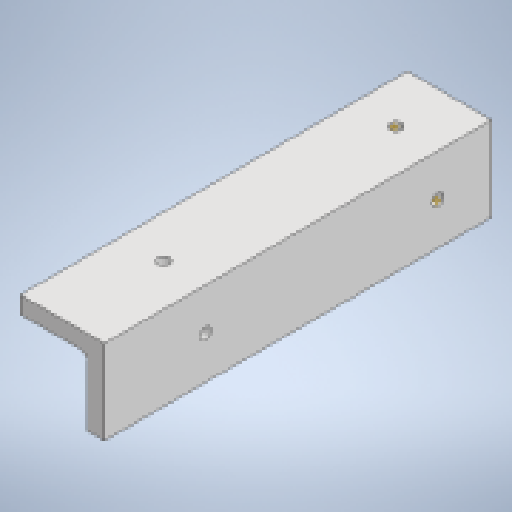
# Autodesk Inventor part: wall-joint
Saved by Autodesk Inventor 2023 (Build 270158000, 158)
## iProperties
Created: 2022-10-04
Part Number: wall-joint
Material: Generic
Document SubType Name: Modeling
Designer: carso
Density: 1 g/cm^3
Appearance: Default
Author: carso
Autodesk Inventor part; units mm, degrees
ref_plane "YZ Plane" through (0, 0, 0) normal (1, 0, 0) x (0, 1, 0)
ref_plane "XZ Plane" through (0, 0, 0) normal (0, 1, 0) x (-1, 0, 0)
ref_plane "XY Plane" through (0, 0, 0) normal (0, 0, 1) x (1, 0, 0)
sketch "Sketch1" plane through (0, 0, 0) normal (0, 1, 0) x (-1, 0, 0)
  line L0 (0, 0) -> (0, 115)
  line L1 (0, 115) -> (5, 115)
  line L2 (0, 0) -> (25, 0)
  line L3 (25, 0) -> (25, 2)
  line L4 (5, 115) -> (5, 0)
  line L5 (25, 2) -> (0, 2)
  line L6 (5, 2) -> (10, 2)
  line L7 (5, 7) -> (5, 2)
  dimension "d1" = 5
  dimension "d2" = 25
  dimension "d3" = 2
  dimension "d60" = 115
  constraints: 16 end point, 4 point on line, 3 perpendicular, 2 horizontal, 2 vertical
  measures "d1" distance of L0.end L1.end
  measures "d2" distance of L0.start L2.end
  measures "d3" distance of L2.end L3.end
  measures "d60" distance of L0.start L0.end
extrude "Extrusion2" add sketch "Sketch1" along normal blind 20
sketch "Sketch3" plane through (0, 20, 0) normal (0, 1, 0) x (1, 0, 0)
  line L0 (0, 0) -> (-25, 0)
  line L1 (-25, 0) -> (-25, -2) projected
  line L2 (-25, 0) -> (-25, -2)
  line L3 (-25, -2) -> (-5, -2)
  line L4 (-5, -115) -> (0, -115) projected
  line L5 (-5, -115) -> (0, -115)
  line L6 (0, 0) -> (-25, 0) projected
  line L7 (0, -115) -> (0, 0)
  line L8 (-5, -115) -> (-25, -115)
  line L9 (-25, -115) -> (-25, -2)
  constraints: 14 end point, 3 perpendicular, 2 collinear, 2 horizontal
extrude "Extrusion3" add sketch "Sketch3" along normal blind 5
fillet "Face Fillet1" radius 2 1 edges at (-5, 10, 2)
fillet "Face Fillet2" radius 2 1 edges at (-16, 20, 2)
hole "Hole3" at (0, 12.5, 15.9996) direction (-1, 0, 0) diameter 3.5 depth 8.8
hole "Hole4" at (-12.5, 25, 16) direction (0, -1, 0) diameter 3.5 depth 8.8
sketch "Sketch11" plane through (0, 25, 0) normal (0, 1, 0) x (1, 0, 0)
  line L0 (-5, -115) -> (0, -115) projected
  line L1 (0, -115) -> (-12.5, -115)
  line L2 (-12.5, -115) -> (-12.5, -85)
  line L3 (-12.5, -85) -> (0, -85)
  line L4 (0, -85) -> (0, -115)
  point P0 (0, 0)
  dimension "d82" = 12.5
  dimension "d83" = 30
  constraints: 8 end point, 2 parallel, 1 horizontal, 1 perpendicular
  measures "d82" distance of L2.end L3.end
  measures "d83" distance of L1.end L2.end
hole "Hole7" at (-12.5, 25, 85) direction (0, -1, 0) diameter 3.5 depth 8.8
sketch "Sketch12" plane through (0, 0, 115) normal (1, 0, 0) x (0, 0, -1)
  line L0 (115, 25) -> (0, 25) projected
  line L1 (0, 25) -> (30, 25)
  line L2 (30, 25) -> (30, 12.5)
  line L3 (30, 12.5) -> (0, 12.5)
  line L4 (0, 12.5) -> (0, 25)
  point P0 (115, 0)
  dimension "d91" = 30
  dimension "d92" = 12.5
  constraints: 8 end point, 2 parallel, 1 horizontal, 1 perpendicular
  measures "d91" distance of L2.end L3.end
  measures "d92" distance of L1.end L2.end
hole "Hole8" at (0, 12.5, 85) direction (-1, 0, 0) diameter 3.5 depth 8.8
body "Solid3"
